Autodesk Inventor part; units mm, degrees
(part 2 of 2)
  spline S240 degree 2 poles (37.9379, -36.8849) (37.6951, -36.6832) (37.4645, -36.1356) (37.4645, -35.831) knots 0 0 0 1 2 2 2
  spline S241 degree 2 poles (37.4645, -35.831) (37.4645, -35.3946) (37.9462, -34.8142) (38.4031, -34.6207) knots 0 0 0 1 2 2 2
  line L284 (38.4031, -34.6207) -> (38.4031, -34.6001)
  spline S242 degree 2 poles (38.4031, -34.6001) (37.9544, -34.3819) (37.6004, -33.7603) (37.6004, -33.3775) knots 0 0 0 1 2 2 2
  spline S243 degree 2 poles (37.6004, -33.3775) (37.6004, -33.0975) (37.8474, -32.6076) (38.0903, -32.4142) knots 0 0 0 1 2 2 2
  spline S244 degree 2 poles (38.0903, -32.4142) (38.3249, -32.2289) (39.0371, -32.0066) (39.4817, -32.0066) knots 0 0 0 1 2 2 2
  spline S245 degree 2 poles (39.4817, -32.0066) (39.951, -32.0066) (40.6508, -32.2083) (40.8773, -32.373) knots 0 0 0 1 2 2 2
  spline S246 degree 2 poles (40.8773, -32.373) (41.1078, -32.5377) (41.3548, -33.0152) (41.3548, -33.291) knots 0 0 0 1 2 2 2
  spline S247 degree 2 poles (41.3548, -33.291) (41.3548, -33.6533) (40.9349, -34.2337) (40.5026, -34.4354) knots 0 0 0 1 2 2 2
  line L285 (40.5026, -34.4354) -> (40.5026, -34.4519)
  spline S248 degree 2 poles (40.5026, -34.4519) (41.009, -34.6578) (41.4865, -35.3247) (41.4865, -35.7898) knots 0 0 0 1 2 2 2
  spline S249 degree 2 poles (40.2268, -35.8434) (40.2268, -35.5922) (40.0128, -35.3288) (39.667, -35.16) knots 0 0 0 1 2 2 2
  spline S250 degree 2 poles (39.667, -35.16) (39.5682, -35.1147) (39.1935, -34.9706) (39.0494, -34.9089) knots 0 0 0 1 2 2 2
  spline S251 degree 2 poles (39.0494, -34.9089) (38.9177, -35.0406) (38.7078, -35.4358) (38.7078, -35.6705) knots 0 0 0 1 2 2 2
  spline S252 degree 2 poles (38.7078, -35.6705) (38.7078, -36.0245) (39.1606, -36.4485) (39.527, -36.4485) knots 0 0 0 1 2 2 2
  spline S253 degree 2 poles (39.527, -36.4485) (39.6299, -36.4485) (39.8851, -36.3826) (39.9839, -36.3168) knots 0 0 0 1 2 2 2
  spline S254 degree 2 poles (39.9839, -36.3168) (40.0951, -36.2386) (40.2268, -36.0245) (40.2268, -35.8434) knots 0 0 0 1 2 2 2
  spline S255 degree 2 poles (40.1157, -33.4392) (40.1157, -33.1799) (39.774, -32.8711) (39.4817, -32.8711) knots 0 0 0 1 2 2 2
  spline S256 degree 2 poles (39.4817, -32.8711) (39.2018, -32.8711) (38.8601, -33.151) (38.8601, -33.3569) knots 0 0 0 1 2 2 2
  spline S257 degree 2 poles (38.8601, -33.3569) (38.8601, -33.5586) (39.0659, -33.8097) (39.2841, -33.9126) knots 0 0 0 1 2 2 2
  spline S258 degree 2 poles (39.2841, -33.9126) (39.3788, -33.962) (39.6423, -34.0649) (39.8604, -34.1473) knots 0 0 0 1 2 2 2
  spline S259 degree 2 poles (39.8604, -34.1473) (39.9922, -33.9744) (40.1157, -33.6492) (40.1157, -33.4392) knots 0 0 0 1 2 2 2
  line L286 (48.7772, -37.2019) -> (48.7772, -35.2876)
  spline S260 degree 2 poles (48.7772, -35.2876) (48.7772, -35.0036) (48.7566, -34.6166) (48.7072, -34.4931) knots 0 0 0 1 2 2 2
  spline S261 degree 2 poles (48.7072, -34.4931) (48.6537, -34.3696) (48.4396, -34.2584) (48.2461, -34.2584) knots 0 0 0 1 2 2 2
  spline S262 degree 2 poles (48.2461, -34.2584) (48.1103, -34.2584) (47.8468, -34.3778) (47.6904, -34.489) knots 0 0 0 1 2 2 2
  line L287 (47.6904, -34.489) -> (47.6904, -37.2019)
  line L288 (47.6904, -37.2019) -> (46.4883, -37.2019)
  line L289 (46.4883, -37.2019) -> (46.4883, -35.2876)
  spline S263 degree 2 poles (46.4883, -35.2876) (46.4883, -35.0077) (46.4636, -34.6166) (46.4142, -34.4931) knots 0 0 0 1 2 2 2
  spline S264 degree 2 poles (46.4142, -34.4931) (46.3607, -34.3696) (46.1466, -34.2584) (45.9531, -34.2584) knots 0 0 0 1 2 2 2
  spline S265 degree 2 poles (45.9531, -34.2584) (45.8091, -34.2584) (45.525, -34.3943) (45.3933, -34.489) knots 0 0 0 1 2 2 2
  line L290 (45.3933, -34.489) -> (45.3933, -37.2019)
  line L291 (45.3933, -37.2019) -> (44.1994, -37.2019)
  line L292 (44.1994, -37.2019) -> (44.1994, -33.3692)
  line L293 (44.1994, -33.3692) -> (45.3933, -33.3692)
  line L294 (45.3933, -33.3692) -> (45.3933, -33.7932)
  spline S266 degree 2 poles (45.3933, -33.7932) (45.6856, -33.5462) (46.2084, -33.2663) (46.5336, -33.2663) knots 0 0 0 1 2 2 2
  spline S267 degree 2 poles (46.5336, -33.2663) (46.8835, -33.2663) (47.4187, -33.5998) (47.5587, -33.9332) knots 0 0 0 1 2 2 2
  spline S268 degree 2 poles (47.5587, -33.9332) (47.9003, -33.6121) (48.5096, -33.2663) (48.8225, -33.2663) knots 0 0 0 1 2 2 2
  spline S269 degree 2 poles (48.8225, -33.2663) (49.0901, -33.2663) (49.5141, -33.4351) (49.6582, -33.608) knots 0 0 0 1 2 2 2
  spline S270 degree 2 poles (49.6582, -33.608) (49.8187, -33.7932) (49.9793, -34.2996) (49.9793, -34.7072) knots 0 0 0 1 2 2 2
  line L295 (49.9793, -34.7072) -> (49.9793, -37.2019)
  line L296 (49.9793, -37.2019) -> (48.7772, -37.2019)
  line L297 (55.438, -37.2019) -> (55.438, -35.2876)
  spline S271 degree 2 poles (55.438, -35.2876) (55.438, -35.0036) (55.4174, -34.6166) (55.368, -34.4931) knots 0 0 0 1 2 2 2
  spline S272 degree 2 poles (55.368, -34.4931) (55.3145, -34.3696) (55.1004, -34.2584) (54.907, -34.2584) knots 0 0 0 1 2 2 2
  spline S273 degree 2 poles (54.907, -34.2584) (54.7711, -34.2584) (54.5076, -34.3778) (54.3512, -34.489) knots 0 0 0 1 2 2 2
  line L298 (54.3512, -34.489) -> (54.3512, -37.2019)
  line L299 (54.3512, -37.2019) -> (53.1491, -37.2019)
  line L300 (53.1491, -37.2019) -> (53.1491, -35.2876)
  spline S274 degree 2 poles (53.1491, -35.2876) (53.1491, -35.0077) (53.1244, -34.6166) (53.075, -34.4931) knots 0 0 0 1 2 2 2
  spline S275 degree 2 poles (53.075, -34.4931) (53.0215, -34.3696) (52.8074, -34.2584) (52.614, -34.2584) knots 0 0 0 1 2 2 2
  spline S276 degree 2 poles (52.614, -34.2584) (52.4699, -34.2584) (52.1858, -34.3943) (52.0541, -34.489) knots 0 0 0 1 2 2 2
  line L301 (52.0541, -34.489) -> (52.0541, -37.2019)
  line L302 (52.0541, -37.2019) -> (50.8602, -37.2019)
  line L303 (50.8602, -37.2019) -> (50.8602, -33.3692)
  line L304 (50.8602, -33.3692) -> (52.0541, -33.3692)
  line L305 (52.0541, -33.3692) -> (52.0541, -33.7932)
  spline S277 degree 2 poles (52.0541, -33.7932) (52.3464, -33.5462) (52.8692, -33.2663) (53.1944, -33.2663) knots 0 0 0 1 2 2 2
  spline S278 degree 2 poles (53.1944, -33.2663) (53.5443, -33.2663) (54.0795, -33.5998) (54.2195, -33.9332) knots 0 0 0 1 2 2 2
  spline S279 degree 2 poles (54.2195, -33.9332) (54.5611, -33.6121) (55.1704, -33.2663) (55.4833, -33.2663) knots 0 0 0 1 2 2 2
  spline S280 degree 2 poles (55.4833, -33.2663) (55.7509, -33.2663) (56.1749, -33.4351) (56.319, -33.608) knots 0 0 0 1 2 2 2
  spline S281 degree 2 poles (56.319, -33.608) (56.4795, -33.7932) (56.6401, -34.2996) (56.6401, -34.7072) knots 0 0 0 1 2 2 2
  line L306 (56.6401, -34.7072) -> (56.6401, -37.2019)
  line L307 (56.6401, -37.2019) -> (55.438, -37.2019)
  point P0 (0, 0)
  dimension "d45" = 8.7721
  dimension "d46" = 40.64
  constraints: 18 end point, 17 horizontal
  measures "d45" distance between parallel lines of L1 L0
  measures "d46" distance between parallel lines of L6 L0
extrude "Extrusion4" cut sketch "Sketch7" against normal blind 2.3813
fillet "Fillet1" radius 1.5875 9 edges at (-55.626, 0, -12.7) (-29.972, 0, -12.7) (-0.889, 0, -12.7) (30.099, 0, -12.7) (38.9043, 0, 19.05) (13.7499, 0, 19.05) (-9.3726, 0, 19.05) (-32.4951, 0, 19.05) (-55.6175, 0, 19.05)
fillet "Fillet2" radius 1.5875 4 edges at (-63.5, -3.175, 44.45) (63.5, -3.175, 44.45) (63.5, -3.175, -44.45) (-63.5, -3.175, -44.45)
equation "\"gap0\" = frontGapBetweenHoles"
equation "\"gap1\" = 0.5 * hex5mmHole + 0.5 * hex4mmHole + frontGapBetweenHoles"
equation "\"gap2\" = 0.5 * hex6mmHole + 0.5 * hex5mmHole + frontGapBetweenHoles"
equation "\"gap3\" = 0.5 * hex7mmHole + 0.5 * hex6mmHole + frontGapBetweenHoles"
equation "\"gap4\" = 0.5 * hex8mmHole + 0.5 * hex7mmHole + frontGapBetweenHoles"
equation "\"gap5\" = backGapBetweenHoles"
equation "\"gap6\" = 0.5 * hex12mmHole + 0.5 * hex10mmHole + backGapBetweenHoles"
equation "\"gap7\" = 0.5 * hex14mmHole + 0.5 * hex12mmHole + backGapBetweenHoles"
equation "\"gap8\" = 0.5 * hex17mmHole + 0.5 * hex14mmHole + backGapBetweenHoles"
equation "\"d46\" = centerLineForBackText"
equation "\"frontGapBetweenHoles\" = 7.88247"
equation "\"backGapBetweenHoles\" = 7.874"
equation "\"centerLineForFrontText\" = 8.3185"
equation "\"centerLineForBackText\" = 40.64"
body "Solid1"
